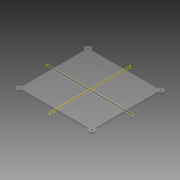
# Autodesk Inventor part: Part1
Saved by Autodesk Inventor 2015 (Build 190159000, 159)
## iProperties
Created: 2014-08-06
Part Number: Part1
Material: PMMA Plastic
Document SubType Name: Modeling
Designer: Patrick Camilleri
Density: 1.188 g/cm^3
Appearance: Polycarbonate - Clear
Author: Patrick Camilleri
Autodesk Inventor part; units mm, degrees
ref_plane "XY Plane" through (0, 0, 0) normal (0, 0, 1) x (1, 0, 0)
sketch "Sketch1" plane through (0, 0, 0) normal (0, 0, 1) x (1, 0, 0)
  line L0 (-116.7, 110) -> (116.7, 110) construction
  line L1 (116.7, 110) -> (116.7, -110) construction
  line L2 (116.7, -110) -> (-116.7, -110) construction
  line L3 (-116.7, -110) -> (-116.7, 110) construction
  line L4 (-116.7, 110) -> (116.7, -110) construction
  line L5 (116.7, 110) -> (-116.7, -110) construction
  line L6 (119.7, 113) -> (-119.7, 113)
  line L7 (-119.7, 113) -> (-119.7, -113)
  line L8 (-119.7, -113) -> (119.7, -113)
  line L9 (119.7, -113) -> (119.7, 113)
  line L10 (-124.7, 118) -> (124.7, 118)
  line L11 (124.7, 118) -> (124.7, -118)
  line L12 (124.7, -118) -> (-124.7, -118)
  line L13 (-124.7, -118) -> (-124.7, 118)
  line L14 (-124.7, -108) -> (-124.7, -118)
  line L15 (-124.7, -118) -> (-114.7, -118)
  arc A0 (-124.7, -108) -> (-114.7, -118) centre (-124.7, -118) ccw
  line L16 (0, -143.5617) -> (0, 172.7629) construction
  line L17 (-168.9533, 0) -> (174.0212, 0) construction
  line L18 (124.7, -108) -> (124.7, -118)
  line L19 (124.7, -118) -> (114.7, -118)
  arc A1 (114.7, -118) -> (124.7, -108) centre (124.7, -118) ccw
  arc A2 (124.7, 108) -> (114.7, 118) centre (124.7, 118) ccw
  line L20 (124.7, 108) -> (124.7, 118)
  line L21 (124.7, 118) -> (114.7, 118)
  line L22 (-124.7, 108) -> (-124.7, 118)
  line L23 (-124.7, 118) -> (-114.7, 118)
  arc A3 (-114.7, 118) -> (-124.7, 108) centre (-124.7, 118) ccw
  circle A4 centre (-124.7, 118) radius 3
  circle A5 centre (124.7, 118) radius 3
  circle A6 centre (-124.7, -118) radius 3
  circle A7 centre (124.7, -118) radius 3
  point P0 (0, 0)
  point P1 (-124.7, 118)
  dimension "d0" = 233.4
  dimension "d1" = 220
  dimension "d2" = 3
  dimension "d3" = 5
  dimension "d8" = 10
  dimension "d9" = 6
  dimension "d10" = 6
  dimension "d11" = 6
  dimension "d12" = 6
  constraints: 48 end point, 13 symmetric about line, 8 centre point, 8 point on circle, 8 point on line, 6 parallel, 4 coincident, 4 perpendicular, 2 horizontal, 2 midpoint, 2 vertical, 9 other
  measures "d0" distance of L1.end L2.end
  measures "d1" distance of L0.end L1.end
  measures "d2" distance between parallel lines of L0 L6
  measures "d3" distance between parallel lines of L6 L10
  measures "d8" distance of L14.start L14.end
  measures "d9" diameter of A4
  measures "d10" diameter of A5
  measures "d11" diameter of A6
  measures "d12" diameter of A7
extrude "Extrusion1" add sketch "Sketch1" along normal blind 6 contours L9 L8 L7 L6 | L13 A4 L10 | L10 A4 L13 | A4 L13 A3 L10 | L10 A5 L11 A7 L12 A6 L13 A4 | A2 L11 A5 L10 | L13 A6 L12 A0 | A5 L11 L10 | L10 L11 A5 | A6 L12 L13 | L13 L12 A6 | A1 L12 A7 L11 | A7 L12 L11 | L11 L12 A7
ref_plane "Work Plane1" through (-131.7711, -125.0711, 6) normal (0, 0, 1) x (1, 0, 0)
sketch "Sketch2" plane through (-131.7711, -125.0711, 6) normal (0, 0, 1) x (1, 0, 0)
  line L0 (246.4711, 243.0711) -> (17.0711, 243.0711) projected
  arc A0 (17.0711, 243.0711) -> (7.0711, 233.0711) centre (7.0711, 243.0711) ccw projected
  line L1 (7.0711, 233.0711) -> (7.0711, 17.0711) projected
  arc A1 (7.0711, 17.0711) -> (17.0711, 7.0711) centre (7.0711, 7.0711) ccw projected
  line L2 (17.0711, 7.0711) -> (246.4711, 7.0711) projected
  arc A2 (246.4711, 7.0711) -> (256.4711, 17.0711) centre (256.4711, 7.0711) ccw projected
  line L3 (256.4711, 17.0711) -> (256.4711, 233.0711) projected
  arc A3 (256.4711, 233.0711) -> (246.4711, 243.0711) centre (256.4711, 243.0711) ccw projected
  circle A4 centre (7.0711, 243.0711) radius 3
  circle A5 centre (256.4711, 243.0711) radius 3
  circle A6 centre (256.4711, 7.0711) radius 3
  circle A7 centre (7.0711, 7.0711) radius 3
  point P0 (131.7711, 125.0711)
  dimension "d15" = 6
  dimension "d16" = 6
  dimension "d17" = 6
  dimension "d18" = 6
  constraints: 4 centre point, 4 coincident
  measures "d15" diameter of A4
  measures "d16" diameter of A5
  measures "d17" diameter of A6
  measures "d18" diameter of A7
extrude "Extrusion2" cut sketch "Sketch2" against normal blind 6 contours A7
mirror "Mirror1" about plane through (0, 0, 0) normal (1, 0, 0) of "Extrusion2"
mirror "Mirror2" about plane through (0, 0, 0) normal (0, 1, 0) of "Extrusion2", "Mirror1"
sketch "Sketch3" plane through (-131.7711, -125.0711, 6) normal (0, 0, 1) x (1, 0, 0)
  circle A0 centre (256.4711, 243.0711) radius 3 projected
  circle A1 centre (7.0711, 243.0711) radius 3 projected
  circle A2 centre (256.4711, 7.0711) radius 3 projected
  circle A3 centre (7.0711, 7.0711) radius 3 projected
  line L0 (246.4711, 243.0711) -> (17.0711, 243.0711) projected
  arc A4 (17.0711, 243.0711) -> (7.0711, 233.0711) centre (7.0711, 243.0711) ccw projected
  line L1 (7.0711, 233.0711) -> (7.0711, 17.0711) projected
  arc A5 (7.0711, 17.0711) -> (17.0711, 7.0711) centre (7.0711, 7.0711) ccw projected
  line L2 (17.0711, 7.0711) -> (246.4711, 7.0711) projected
  arc A6 (246.4711, 7.0711) -> (256.4711, 17.0711) centre (256.4711, 7.0711) ccw projected
  line L3 (256.4711, 17.0711) -> (256.4711, 233.0711) projected
  arc A7 (256.4711, 233.0711) -> (246.4711, 243.0711) centre (256.4711, 243.0711) ccw projected
  line L4 (12.0711, 238.0711) -> (251.4711, 12.0711) construction
  line L5 (251.4711, 238.0711) -> (12.0711, 12.0711) construction
  line L6 (249.9711, 236.4371) -> (13.5711, 236.4371) construction
  line L7 (13.5711, 236.4371) -> (13.5711, 13.7051) construction
  line L8 (13.5711, 13.7051) -> (249.9711, 13.7051) construction
  line L9 (249.9711, 13.7051) -> (249.9711, 236.4371) construction
  line L10 (12.0711, 135.0711) -> (15.0711, 115.0711) construction
  line L11 (15.0711, 135.0711) -> (12.0711, 115.0711) construction
  line L12 (12.0711, 53.7051) -> (15.0711, 53.7051)
  line L13 (15.0711, 53.7051) -> (15.0711, 33.7051)
  line L14 (15.0711, 33.7051) -> (12.0711, 33.7051)
  line L15 (12.0711, 33.7051) -> (12.0711, 53.7051)
  line L16 (12.0711, 37.5309) -> (15.0711, 17.5309) construction
  line L17 (15.0711, 37.5309) -> (12.0711, 17.5309) construction
  point P0 (131.7711, 125.0711)
  point P1 (13.5711, 125.0711)
  point P2 (13.5711, 27.5309)
  dimension "d27" = 3
  dimension "d28" = 20
  dimension "d31" = 3
  dimension "d32" = 20
  dimension "d33" = 20
  constraints: 28 end point, 7 midpoint, 4 parallel, 2 perpendicular, 1 horizontal, 1 point on line
  measures "d27" distance of L10.end L11.end
  measures "d28" distance of L11.start L10.end
  measures "d31" distance of L13.end L14.end
  measures "d32" distance of L12.end L13.end
  measures "d33" distance between parallel lines of L14 L8
extrude "Extrusion3" [suppressed]
mirror "Mirror3" [suppressed]
body "Solid1"
